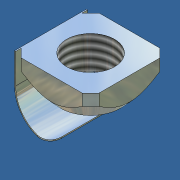
# Autodesk Inventor part: 21.1351/2
Saved by Autodesk Inventor 2012 (Build 160160000, 160)
## iProperties
Created: 2006-12-22
Part Number: 21.1351/2
Document SubType Name: Modeling
Designer: Andy Moles
Material: Steel, Mild
Density: 7.86 g/cm^3
Mass: 4.2544 g
Surface Area: 8.34272 cm^2
Volume: 0.541273 cm^3
Description: M8 SQUARE NUT POS FXG
Vendor: S
Title: M8 SQUARE NUT POS FXG
Author: Andy Moles
Autodesk Inventor part; units mm, degrees
ref_plane "YZ Plane" through (0, 0, 0) normal (1, 0, 0) x (0, 1, 0)
ref_plane "XZ Plane" through (0, 0, 0) normal (0, 1, 0) x (-1, 0, 0)
sketch "Sketch2" plane through (0, 0, 0) normal (0, 0, 1) x (1, 0, 0)
  line L0 (-5.0858, -6.5) -> (5.0858, -6.5)
  line L1 (6.5, -5.0858) -> (6.5, 5.0858)
  line L2 (5.0858, 6.5) -> (-5.0858, 6.5)
  line L3 (-6.5, 5.0858) -> (-6.5, -5.0858)
  line L4 (-6.5, 6.5) -> (6.5, -6.5) construction
  circle A0 centre (0, 0) radius 4
  line L5 (5.0858, 6.5) -> (6.5, 5.0858)
  line L6 (0, -6.5) -> (0, 6.5) construction
  line L7 (-6.5, 0) -> (6.5, 0) construction
  line L8 (-5.0858, 6.5) -> (-6.5, 5.0858)
  line L9 (5.0858, -6.5) -> (6.5, -5.0858)
  line L10 (-5.0858, -6.5) -> (-6.5, -5.0858)
  dimension "THREAD" = 8
  dimension "d3" = 45
  dimension "d4" = 2
  constraints: 22 end point, 6 symmetric about line, 4 parallel, 3 midpoint, 2 coincident, 2 perpendicular, 1 centre point, 1 horizontal
  measures "THREAD" diameter of A0
  measures "d3" angle of L2 L5
  measures "d4" distance of L2.start L1.end
extrude "Extrusion1" add sketch "Sketch2" against normal blind 5.5
ref_plane "Work Plane1" through (-5.7929, -5.7929, -5.5) normal (0.7071068, -0.7071068, 0) x (0.7071068, 0.7071068, 0)
sketch "Sketch4" plane through (-5.7929, -5.7929, -5.5) normal (0.7071068, -0.7071068, 0) x (0.7071068, 0.7071068, 0)
  line L0 (12.1924, 0) -> (4.1924, 0) projected
  line L1 (8.1924, 0) -> (13.1924, 0)
  line L2 (16.3848, 5.5) -> (16.3848, 3.5)
  line L3 (13.1924, 0) -> (16.7968, 3.9518)
  line L4 (13.1924, 0) -> (16.3848, 0)
  line L5 (16.3848, 3.5) -> (16.3848, 0)
  line L6 (16.7968, 3.9518) -> (16.7968, -0.4121)
  line L7 (16.7968, -0.4121) -> (13.1924, -0.4121)
  line L8 (13.1924, -0.4121) -> (13.1924, 0)
  line L9 (8.1924, 5.5) -> (8.1924, 0)
  line L10 (16.3848, 5.5) -> (16.3848, 0) projected
  line L11 (16.3848, 3.5) -> (17.5015, 3.5) construction
  line L12 (9.1924, 5.5) -> (16.3848, 5.5) construction
  dimension "d10" = 5
  dimension "d15" = 2
  constraints: 20 end point, 6 perpendicular, 1 collinear, 1 midpoint, 1 parallel, 1 point on line
  measures "d10" distance of L1.start L1.end
  measures "d15" distance between parallel lines of L11 L12
revolve "Revolution1" cut sketch "Sketch4" angle 360 about axis through (0, 0, 0) along (0, 0, -1)
thread "Thread1" size "M8x1.25" class "6H" standard "ANSI Metric M Profile" full length
sketch "Sketch6" plane through (-3.5464, 0, 2.5351) normal (0, 1, 0) x (-1, 0, 0)
  line L0 (2.9536, -2.5351) -> (2.9536, 6.0056)
  line L1 (2.9536, -2.5351) -> (2.9536, -7.5351)
  arc A0 (-2.6464, -13.1351) -> (2.9536, -7.5351) centre (-2.4158, -7.7657) ccw
  line L2 (2.9536, -2.5351) -> (3.1536, -2.5351)
  line L3 (3.1536, -2.5351) -> (3.1536, -7.5351)
  line L4 (-2.6464, -13.1351) -> (-2.6464, -13.3351)
  arc A1 (-2.6464, -13.3351) -> (3.1536, -7.5351) centre (-2.4158, -7.7657) ccw
  line L5 (2.9536, 0) -> (2.9536, -1.9333)
  line L6 (-5.0858, -2.5351) -> (5.0858, -2.5351)
  line L7 (-8.6322, -2.5351) -> (1.5394, -2.5351) projected
  line L8 (2.9536, -2.5351) -> (2.9536, -4.4684) projected
  point P0 (0, 0)
  point P1 (-15.0649, 7.0019)
  dimension "d25" = 5
  dimension "d23" = 0.2
  dimension "d22" = 0.2
  dimension "d21" = 10.8
  dimension "d24" = 5.3743
  constraints: 12 end point, 4 point on circle, 3 collinear, 2 centre point, 2 horizontal, 2 parallel, 2 perpendicular, 1 coincident, 3 other
  measures "d25" distance of L0.start L1.end
  measures "d23" distance of L0.start L2.end
  measures "d22" distance of L4.start L4.end
  measures "d21" distance from line of L4.end L2
  measures "d24" radius of A0
extrude "Extrusion3" add sketch "Sketch6" along normal mid plane 12
fillet "Fillet2" radius 2 2 edges at (-0.9, -6, -10.7) (-0.9, 6, -10.7)
body "Solid1"
